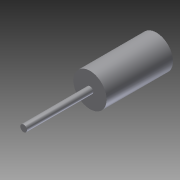
# Autodesk Inventor part: 110V Motor
Saved by Autodesk Inventor 2012 (Build 160160000, 160)
## iProperties
Created: 2011-08-19
Part Number: 110V Motor
Material: Default
Document SubType Name: Modeling
Designer: Minh Tran
Density: 1 g/cm^3
Author: Minh Tran
Autodesk Inventor part; units mm, degrees
ref_plane "YZ Plane" through (0, 0, 0) normal (1, 0, 0) x (0, 1, 0)
ref_plane "XZ Plane" through (0, 0, 0) normal (0, 1, 0) x (-1, 0, 0)
ref_plane "XY Plane" through (0, 0, 0) normal (0, 0, 1) x (1, 0, 0)
sketch "Sketch1" plane through (0, 0, 0) normal (0, 0, 1) x (1, 0, 0)
  circle A0 centre (0, 0) radius 63.5
  dimension "d0" = 127
  constraints: 1 centre point, 1 coincident
  measures "d0" diameter of A0
extrude "Extrusion1" add sketch "Sketch1" along normal blind 254
sketch "Sketch2" plane through (0, 0, 254) normal (0, 0, 1) x (1, 0, 0)
  circle A0 centre (0, 0) radius 63.5 projected
  circle A1 centre (0, 0) radius 12.7
  dimension "d3" = 25.4
  constraints: 1 centre point, 1 coincident
  measures "d3" diameter of A1
extrude "Extrusion2" add sketch "Sketch2" along normal blind 254 contours A1
body "Solid1"
